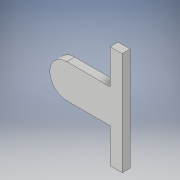
# Autodesk Inventor part: Air Restricter 1.1
Saved by Autodesk Inventor 2019 (Build 230136000, 136)
## iProperties
Created: 2019-04-01
Part Number: Air Restricter 1.1
Material: Generic
Document SubType Name: Modeling
Designer: Kepler
Density: 1 g/cm^3
Appearance: Default
Author: Kepler
Autodesk Inventor part; units mm, degrees
ref_plane "YZ Plane" through (0, 0, 0) normal (1, 0, 0) x (0, 1, 0)
ref_plane "XZ Plane" through (0, 0, 0) normal (0, 1, 0) x (-1, 0, 0)
ref_plane "XY Plane" through (0, 0, 0) normal (0, 0, 1) x (1, 0, 0)
sketch "Sketch1" plane through (0, 0, 0) normal (0, 0, 1) x (1, 0, 0)
  arc A0 (0, 9.75) -> (0, -9.75) centre (0, 0) ccw
  line L0 (0, 9.75) -> (25, 9.75)
  line L1 (25, -9.75) -> (0, -9.75)
  line L2 (25, 9.75) -> (25, 29.75)
  line L3 (25, 29.75) -> (32, 29.75)
  line L4 (32, 29.75) -> (32, 9.75)
  line L5 (32, 9.75) -> (32, -9.75)
  line L6 (32, -9.75) -> (32, -29.75)
  line L7 (32, -29.75) -> (25, -29.75)
  line L8 (25, -29.75) -> (25, -9.75)
  dimension "d0" = 19.5
  dimension "d1" = 25
  dimension "d4" = 20
  dimension "d5" = 7
  dimension "d6" = 20
  dimension "d7" = 59.5
  dimension "d8" = 20
  constraints: 18 end point, 4 perpendicular, 3 point on line, 2 point on circle, 2 tangent, 1 centre point, 1 coincident, 1 horizontal, 1 parallel, 1 vertical
  measures "d0" diameter of A0
  measures "d1" distance of L0.start L0.end
  measures "d4" distance of L0.end L2.end
  measures "d5" distance of L2.end L3.end
  measures "d6" distance of L5.end L6.end
  measures "d7" distance between parallel lines of L7 L3
  measures "d8" distance from line of L4.end L3
extrude "Extrusion1" add sketch "Sketch1" along normal blind 4.6
body "Solid1"
